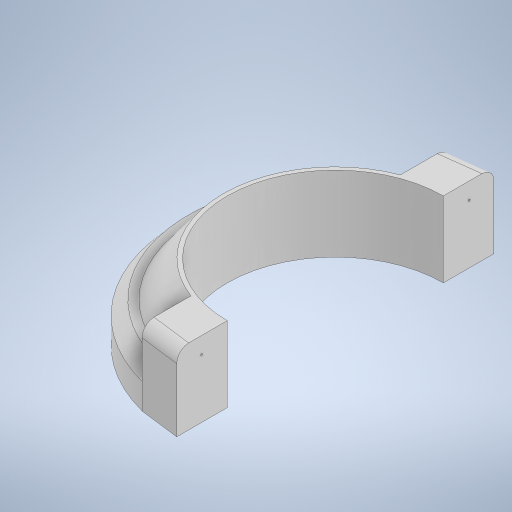
# Autodesk Inventor part: 2_Obrecz_kolanko
Saved by Autodesk Inventor 2024 (Build 280153000, 153)
## iProperties
Created: 2023-12-16
Part Number: 2_Obrecz_kolanko
Material: Generic
Document SubType Name: Modeling
Designer: Piter
Density: 1 g/cm^3
Appearance: Default
Author: Piter
Autodesk Inventor part; units mm, degrees
ref_plane "YZ Plane" through (0, 0, 0) normal (1, 0, 0) x (0, 1, 0)
ref_plane "XZ Plane" through (0, 0, 0) normal (0, 1, 0) x (-1, 0, 0)
ref_plane "XY Plane" through (0, 0, 0) normal (0, 0, 1) x (1, 0, 0)
sketch "Sketch1" plane through (0, 0, 0) normal (0, 1, 0) x (-1, 0, 0)
  circle A0 centre (0, 0) radius 27.25
  circle A1 centre (0, 0) radius 40
  line L0 (0, 40) -> (0, -40)
  line L1 (0, 27.25) -> (0, 40)
  line L2 (0, 0) -> (45.8367, 0)
  line L3 (0, -27.25) -> (0, -40)
  circle A2 centre (0, 0) radius 35
  line L4 (0, -27.25) -> (10, -27.25)
  line L5 (10, -27.25) -> (10, -40)
  line L6 (10, -40) -> (0, -40)
  line L7 (0, -40) -> (0, -27.25)
  line L8 (0, 27.25) -> (10, 27.25)
  line L9 (10, 27.25) -> (10, 40)
  line L10 (10, 40) -> (0, 40)
  point P0 (0, -26.75)
  point P1 (0, 35)
  point P2 (0, -35)
  point P3 (10, -33.541)
  point P4 (10, 38.7298)
  point P5 (10, 33.541)
  dimension "d0" = 54.5
  dimension "d1" = 80
  dimension "d15" = 70
  dimension "d18" = 10
  constraints: 22 end point, 5 symmetric about line, 3 coincident, 2 centre point, 2 horizontal, 2 parallel, 2 point on circle, 1 perpendicular, 1 point on line, 1 vertical, 3 other
  measures "d1" diameter of A1
  measures "d15" diameter of A2
  measures "d18" distance of L5.end L6.end
extrude "Extrusion6" add sketch "Sketch1" along normal blind 10 contours A2 L9 A1 L2 | L2 A1 L5 A2 | L0 A1 L9 A2 | A2 L5 A1 L0
extrude "Extrusion7" add sketch "Sketch1" along normal blind 19 contours L2 A2 L5 L4 A0 | A0 L8 L9 A2 L2 | L0 A2 L9 L8 | L4 L5 A2 L0 | L0 A1 L9 A2 | A2 L5 A1 L0 | L10 L9 A1 | A1 L5 L6
chamfer "Chamfer1" distance 10 distance2 1.25 1 edges at (-10, 9.5, -40) measured on face at (-9.5, 9.5, -40)
chamfer "Chamfer2" distance 1.25 distance2 10 1 edges at (-10, 9.5, 40) measured on face at (-10, 9.5, 39.5)
chamfer "Chamfer3" distance 6.75 distance2 9 1 edges at (-35, 19, 0) measured on face at (-34.5, 19, 0)
chamfer "Chamfer4" distance 3 distance2 3.5 1 edges at (-40, 10, 0) measured on face at (-39.5, 10, 0)
fillet "Fillet1" radius 3 4 edges at (-5, 19, 39.3751) (0, 19, 40) (-5, 19, -39.3751) (0, 19, -40)
sketch "Sketch3" plane through (-10, 0, -38.7298) normal (-1, 0, 0) x (0, 0, 1)
  line L0 (-0.0202, 0) -> (-0.0202, 16) projected
  line L1 (-0.0202, 14.7921) -> (4.9798, 14.7921)
  line L2 (4.9798, 14.7921) -> (4.9798, 19.7921)
  circle A0 centre (4.9798, 14.7921) radius 0.25
  point P0 (38.7298, 0)
  dimension "d32" = 5
  dimension "d33" = 5
  dimension "d34" = 0.5
  constraints: 4 end point, 1 centre point, 1 coincident, 1 horizontal, 1 perpendicular, 1 point on line
  measures "d32" distance of L1.start L1.end
  measures "d33" distance of L1.end L2.end
  measures "d34" diameter of A0
extrude "Extrusion8" cut sketch "Sketch3" against normal through all
mirror "Mirror1" about plane through (0, 0, 0) normal (0, 0, 1) of "Extrusion8"
body "Solid5"
